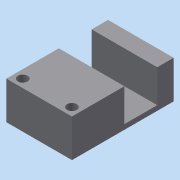
# Autodesk Inventor part: rail mount
Saved by Autodesk Inventor 2015 (Build 190159000, 159)
## iProperties
Created: 2016-06-25
Part Number: rail mount
Material: Generic
Document SubType Name: Modeling
Designer: Dustin
Density: 1 g/cm^3
Appearance: Default
Author: Dustin
Autodesk Inventor part; units mm, degrees
ref_plane "YZ Plane" through (0, 0, 0) normal (1, 0, 0) x (0, 1, 0)
ref_plane "XZ Plane" through (0, 0, 0) normal (0, 1, 0) x (-1, 0, 0)
ref_plane "XY Plane" through (0, 0, 0) normal (0, 0, 1) x (1, 0, 0)
sketch "Sketch1" plane through (0, 0, 0) normal (0, 0, 1) x (1, 0, 0)
  line L0 (0, 0) -> (40, 0)
  line L1 (40, 0) -> (40, 10)
  line L2 (40, 10) -> (0, 10)
  line L3 (0, 10) -> (0, 0)
  dimension "d0" = 40
  dimension "d1" = 10
  constraints: 8 end point, 2 parallel, 1 horizontal, 1 perpendicular
  measures "d0" distance of L1.end L2.end
  measures "d1" distance of L2.end L0.start
extrude "Extrusion1" add sketch "Sketch1" along normal blind 10
sketch "Sketch2" plane through (0, 0, 10) normal (0, 0, 1) x (1, 0, 0)
  line L0 (0, 10) -> (0, 0) projected
  line L1 (40, 10) -> (0, 10) projected
  point P0 (5, 5)
  point P1 (35, 5)
  dimension "d4" = 30
  dimension "d5" = 5
  dimension "d6" = 5
  dimension "d7" = 5
  measures "d4" distance of point (35, 5) point (5, 5)
  measures "d5" distance from line of L0 point (5, 5)
  measures "d6" distance from line of L1 point (5, 5)
  measures "d7" distance from line of L1 point (35, 5)
hole "Hole1" at (5, 5, 10) at (35, 5, 10) direction (0, 0, -1) diameter 6 depth 5 tip angle 118
sketch "Sketch3" plane through (0, 0, 0) normal (0, 0, -1) x (-1, 0, 0)
  line L0 (0, 0) -> (-40, 0) projected
  line L1 (0, 10) -> (0, 0) projected
  line L2 (-40, 10) -> (0, 10) projected
  line L3 (-40, 0) -> (-40, 10) projected
extrude "Extrusion2" add sketch "Sketch3" along normal blind 10
sketch "Sketch4" plane through (0, 0, 10) normal (0, -1, 0) x (1, 0, 0)
  line L0 (40, -20) -> (0, -20)
  line L1 (0, -20) -> (0, -23)
  line L2 (0, -23) -> (40, -23)
  line L3 (40, -23) -> (40, -20)
  point P0 (0, -10)
  dimension "d17" = 3
  constraints: 8 end point, 2 parallel, 1 horizontal, 1 perpendicular
  measures "d17" distance of L0.end L1.end
extrude "Extrusion3" add sketch "Sketch4" against normal blind 52
sketch "Sketch5" plane through (40, 0, -13) normal (0, 0, -1) x (-1, 0, 0)
  line L0 (0, 52) -> (40, 52)
  line L1 (40, 52) -> (40, 62)
  line L2 (40, 62) -> (0, 62)
  line L3 (0, 62) -> (0, 52)
  point P0 (40, 0)
  dimension "d20" = 10
  constraints: 8 end point, 2 parallel, 1 horizontal, 1 perpendicular
  measures "d20" distance of L2.end L0.start
extrude "Extrusion4" add sketch "Sketch5" against normal up to surface (23 mm away)
sketch "Sketch6" plane through (0, 10, 10) normal (0, 1, 0) x (1, 0, 0)
  line L0 (0, 20) -> (0, 0) projected
  line L1 (40, 0) -> (0, 0) projected
  line L2 (40, 20) -> (40, 0) projected
  line L3 (0, 20) -> (40, 20) projected
  point P0 (0, 10)
extrude "Extrusion5" add sketch "Sketch6" along normal blind 22
body "Solid1"
